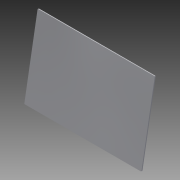
# Autodesk Inventor part: Panel_bottom
Saved by Autodesk Inventor 2013 (Build 170138000, 138)
## iProperties
Created: 2013-01-27
Part Number: Panel_bottom
Material: Aluminum
Document SubType Name: Modeling
Designer: xylzlyx
Density: 1 g/cm^3
Author: xylzlyx
Autodesk Inventor part; units mm, degrees
ref_plane "YZ Plane" through (0, 0, 0) normal (1, 0, 0) x (0, 1, 0)
ref_plane "XZ Plane" through (0, 0, 0) normal (0, 1, 0) x (-1, 0, 0)
ref_plane "XY Plane" through (0, 0, 0) normal (0, 0, 1) x (1, 0, 0)
sketch "ProjectedEdgesBase" plane through (187.5, -125, -3) normal (0, -0.1736482, -0.9848078) x (-1, 0, 0)
  line L0 (0, 244.2323) -> (0, 1.9696)
  line L1 (373, 246.2019) -> (2, 246.2019)
  line L2 (375, 1.9696) -> (375, 244.2323)
  line L3 (2, -0.5209) -> (373, -0.5209)
  line L4 (375, 246.2019) -> (0, 246.2019)
  line L5 (0, 246.2019) -> (0, -0.5209)
  line L6 (0, -0.5209) -> (375, -0.5209)
  line L7 (375, -0.5209) -> (375, 246.2019)
  point P0 (187.5, 122.58)
  point P1 (187.5, 246.2019)
  point P2 (187.5, 246.2019)
  point P3 (187.5, -0.5209)
  point P4 (187.5, -0.5209)
  point P5 (375, 122.8405)
  point P6 (375, 123.101)
  point P7 (0, 122.8405)
  point P8 (0, 123.101)
extrude "BottomPanelExtrusion" add sketch "ProjectedEdgesBase" along normal blind 3
fillet "CornerFillet" radius 2 4 edges at (-187.5, 117.2011, -47.2297) (187.5, 117.2011, -47.2297) (-187.5, -125.7735, -4.3868) (187.5, -125.7735, -4.3868)
